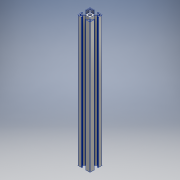
# Autodesk Inventor part: 3030 Extrusion - Y
Saved by Autodesk Inventor 2016 (Build 200138000, 138)
## iProperties
Created: 2016-12-24
Part Number: 3030 Extrusion - Y
Material: Aluminum 6061
Document SubType Name: Modeling
Designer: Scott
Mass: 352.135 g
Surface Area: 1477.59 cm^2
Volume: 130.42 cm^3
Density: 2.7 g/cm^3
Appearance: Aluminum - Flat
Author: Scott
Autodesk Inventor part; units mm, degrees
ref_plane "YZ Plane" through (0, 0, 0) normal (1, 0, 0) x (0, 1, 0)
ref_plane "XZ Plane" through (0, 0, 0) normal (0, 1, 0) x (-1, 0, 0)
ref_plane "XY Plane" through (0, 0, 0) normal (0, 0, 1) x (1, 0, 0)
sketch "Sketch1" plane through (0, 0, 0) normal (0, 0, 1) x (1, 0, 0)
  line L0 (1.9798, -0.0606) -> (9.8798, -0.0606)
  line L1 (20.0798, -0.0606) -> (27.9798, -0.0606)
  arc A0 (-0.0202, 1.9394) -> (1.9798, -0.0606) centre (1.9798, 1.9394) ccw
  line L2 (29.9798, 1.9394) -> (29.9798, 9.8394)
  arc A1 (27.9798, -0.0606) -> (29.9798, 1.9394) centre (27.9798, 1.9394) ccw
  line L3 (29.9798, 20.0394) -> (29.9798, 27.9394)
  arc A2 (29.9798, 27.9394) -> (27.9798, 29.9394) centre (27.9798, 27.9394) ccw
  line L4 (27.9798, 29.9394) -> (20.0798, 29.9394)
  line L5 (9.8798, 29.9394) -> (1.9798, 29.9394)
  line L6 (-0.0202, 27.9394) -> (-0.0202, 20.0394)
  line L7 (-0.0202, 9.8394) -> (-0.0202, 1.9394)
  arc A3 (1.9798, 29.9394) -> (-0.0202, 27.9394) centre (1.9798, 27.9394) ccw
  circle A4 centre (14.9798, 14.9394) radius 3.4
  line L8 (24.9798, 1.4394) -> (27.9798, 1.4394)
  arc A5 (27.9798, 1.4394) -> (28.4798, 1.9394) centre (27.9798, 1.9394) ccw
  line L9 (28.4798, 1.9394) -> (28.4798, 4.9394)
  arc A6 (28.4798, 4.9394) -> (27.9798, 5.4394) centre (27.9798, 4.9394) ccw
  line L10 (29.2298, 9.8394) -> (29.2298, 10.8394)
  line L11 (29.2298, 19.0394) -> (29.2298, 20.0394)
  line L12 (28.4798, 7.1894) -> (28.4798, 10.8394)
  arc A7 (27.9798, 6.6894) -> (28.4798, 7.1894) centre (27.9798, 7.1894) ccw
  line L13 (28.4798, 19.0394) -> (28.4798, 22.6894)
  arc A8 (28.4798, 22.6894) -> (27.9798, 23.1894) centre (27.9798, 22.6894) ccw
  line L14 (20.9262, 19.8252) -> (24.144, 23.0429)
  arc A9 (24.4975, 23.1894) -> (24.144, 23.0429) centre (24.4975, 22.6894) ccw
  line L15 (20.9262, 10.0536) -> (24.144, 6.8358)
  arc A10 (20.7798, 10.4071) -> (20.9262, 10.0536) centre (21.2798, 10.4071) ccw
  line L16 (24.4975, 6.6894) -> (27.9798, 6.6894)
  arc A11 (24.144, 6.8358) -> (24.4975, 6.6894) centre (24.4975, 7.1894) ccw
  line L17 (24.4975, 23.1894) -> (27.9798, 23.1894)
  line L18 (28.4798, 10.8394) -> (29.2298, 10.8394)
  line L19 (28.4798, 19.0394) -> (29.2298, 19.0394)
  line L20 (29.2298, 9.8394) -> (29.9798, 9.8394)
  line L21 (29.2298, 20.0394) -> (29.9798, 20.0394)
  line L22 (20.7798, 10.4071) -> (20.7798, 19.4716)
  arc A12 (20.9262, 19.8252) -> (20.7798, 19.4716) centre (21.2798, 19.4716) ccw
  line L23 (24.4798, 1.9394) -> (24.4798, 4.9394)
  arc A13 (24.4798, 1.9394) -> (24.9798, 1.4394) centre (24.9798, 1.9394) ccw
  line L24 (24.9798, 5.4394) -> (27.9798, 5.4394)
  arc A14 (24.9798, 5.4394) -> (24.4798, 4.9394) centre (24.9798, 4.9394) ccw
  line L25 (28.4798, 24.9394) -> (28.4798, 27.9394)
  arc A15 (28.4798, 27.9394) -> (27.9798, 28.4394) centre (27.9798, 27.9394) ccw
  line L26 (27.9798, 28.4394) -> (24.9798, 28.4394)
  arc A16 (24.9798, 28.4394) -> (24.4798, 27.9394) centre (24.9798, 27.9394) ccw
  line L27 (20.0798, 29.1894) -> (19.0798, 29.1894)
  line L28 (10.8798, 29.1894) -> (9.8798, 29.1894)
  line L29 (22.7298, 28.4394) -> (19.0798, 28.4394)
  arc A17 (23.2298, 27.9394) -> (22.7298, 28.4394) centre (22.7298, 27.9394) ccw
  line L30 (10.8798, 28.4394) -> (7.2298, 28.4394)
  arc A18 (7.2298, 28.4394) -> (6.7298, 27.9394) centre (7.2298, 27.9394) ccw
  line L31 (10.094, 20.8858) -> (6.8762, 24.1036)
  arc A19 (6.7298, 24.4571) -> (6.8762, 24.1036) centre (7.2298, 24.4571) ccw
  line L32 (19.8656, 20.8858) -> (23.0833, 24.1036)
  arc A20 (19.512, 20.7394) -> (19.8656, 20.8858) centre (19.512, 21.2394) ccw
  line L33 (23.2298, 24.4571) -> (23.2298, 27.9394)
  arc A21 (23.0833, 24.1036) -> (23.2298, 24.4571) centre (22.7298, 24.4571) ccw
  line L34 (6.7298, 24.4571) -> (6.7298, 27.9394)
  line L35 (19.0798, 28.4394) -> (19.0798, 29.1894)
  line L36 (10.8798, 28.4394) -> (10.8798, 29.1894)
  line L37 (20.0798, 29.1894) -> (20.0798, 29.9394)
  line L38 (9.8798, 29.1894) -> (9.8798, 29.9394)
  line L39 (19.512, 20.7394) -> (10.4475, 20.7394)
  arc A22 (10.094, 20.8858) -> (10.4475, 20.7394) centre (10.4475, 21.2394) ccw
  line L40 (27.9798, 24.4394) -> (24.9798, 24.4394)
  arc A23 (27.9798, 24.4394) -> (28.4798, 24.9394) centre (27.9798, 24.9394) ccw
  line L41 (24.4798, 24.9394) -> (24.4798, 27.9394)
  arc A24 (24.4798, 24.9394) -> (24.9798, 24.4394) centre (24.9798, 24.9394) ccw
  line L42 (4.9798, 28.4394) -> (1.9798, 28.4394)
  arc A25 (1.9798, 28.4394) -> (1.4798, 27.9394) centre (1.9798, 27.9394) ccw
  line L43 (1.4798, 27.9394) -> (1.4798, 24.9394)
  arc A26 (1.4798, 24.9394) -> (1.9798, 24.4394) centre (1.9798, 24.9394) ccw
  line L44 (0.7298, 20.0394) -> (0.7298, 19.0394)
  line L45 (0.7298, 10.8394) -> (0.7298, 9.8394)
  line L46 (1.4798, 22.6894) -> (1.4798, 19.0394)
  arc A27 (1.9798, 23.1894) -> (1.4798, 22.6894) centre (1.9798, 22.6894) ccw
  line L47 (1.4798, 10.8394) -> (1.4798, 7.1894)
  arc A28 (1.4798, 7.1894) -> (1.9798, 6.6894) centre (1.9798, 7.1894) ccw
  line L48 (9.0333, 10.0536) -> (5.8156, 6.8358)
  arc A29 (5.462, 6.6894) -> (5.8156, 6.8358) centre (5.462, 7.1894) ccw
  line L49 (9.0333, 19.8252) -> (5.8156, 23.0429)
  arc A30 (9.1798, 19.4716) -> (9.0333, 19.8252) centre (8.6798, 19.4716) ccw
  line L50 (5.462, 23.1894) -> (1.9798, 23.1894)
  arc A31 (5.8156, 23.0429) -> (5.462, 23.1894) centre (5.462, 22.6894) ccw
  line L51 (5.462, 6.6894) -> (1.9798, 6.6894)
  line L52 (1.4798, 19.0394) -> (0.7298, 19.0394)
  line L53 (1.4798, 10.8394) -> (0.7298, 10.8394)
  line L54 (0.7298, 20.0394) -> (-0.0202, 20.0394)
  line L55 (0.7298, 9.8394) -> (-0.0202, 9.8394)
  line L56 (9.1798, 19.4716) -> (9.1798, 10.4071)
  arc A32 (9.0333, 10.0536) -> (9.1798, 10.4071) centre (8.6798, 10.4071) ccw
  line L57 (5.4798, 27.9394) -> (5.4798, 24.9394)
  arc A33 (5.4798, 27.9394) -> (4.9798, 28.4394) centre (4.9798, 27.9394) ccw
  line L58 (4.9798, 24.4394) -> (1.9798, 24.4394)
  arc A34 (4.9798, 24.4394) -> (5.4798, 24.9394) centre (4.9798, 24.9394) ccw
  line L59 (1.4798, 4.9394) -> (1.4798, 1.9394)
  arc A35 (1.4798, 1.9394) -> (1.9798, 1.4394) centre (1.9798, 1.9394) ccw
  line L60 (1.9798, 1.4394) -> (4.9798, 1.4394)
  arc A36 (4.9798, 1.4394) -> (5.4798, 1.9394) centre (4.9798, 1.9394) ccw
  line L61 (9.8798, 0.6894) -> (10.8798, 0.6894)
  line L62 (19.0798, 0.6894) -> (20.0798, 0.6894)
  line L63 (7.2298, 1.4394) -> (10.8798, 1.4394)
  arc A37 (6.7298, 1.9394) -> (7.2298, 1.4394) centre (7.2298, 1.9394) ccw
  line L64 (19.0798, 1.4394) -> (22.7298, 1.4394)
  arc A38 (22.7298, 1.4394) -> (23.2298, 1.9394) centre (22.7298, 1.9394) ccw
  line L65 (19.8656, 8.9929) -> (23.0833, 5.7752)
  arc A39 (23.2298, 5.4216) -> (23.0833, 5.7752) centre (22.7298, 5.4216) ccw
  line L66 (10.094, 8.9929) -> (6.8762, 5.7752)
  arc A40 (10.4475, 9.1394) -> (10.094, 8.9929) centre (10.4475, 8.6394) ccw
  line L67 (6.7298, 5.4216) -> (6.7298, 1.9394)
  arc A41 (6.8762, 5.7752) -> (6.7298, 5.4216) centre (7.2298, 5.4216) ccw
  line L68 (23.2298, 5.4216) -> (23.2298, 1.9394)
  line L69 (10.8798, 1.4394) -> (10.8798, 0.6894)
  line L70 (19.0798, 1.4394) -> (19.0798, 0.6894)
  line L71 (9.8798, 0.6894) -> (9.8798, -0.0606)
  line L72 (20.0798, 0.6894) -> (20.0798, -0.0606)
  line L73 (10.4475, 9.1394) -> (19.512, 9.1394)
  arc A42 (19.8656, 8.9929) -> (19.512, 9.1394) centre (19.512, 8.6394) ccw
  line L74 (1.9798, 5.4394) -> (4.9798, 5.4394)
  arc A43 (1.9798, 5.4394) -> (1.4798, 4.9394) centre (1.9798, 4.9394) ccw
  line L75 (5.4798, 4.9394) -> (5.4798, 1.9394)
  arc A44 (5.4798, 4.9394) -> (4.9798, 5.4394) centre (4.9798, 4.9394) ccw
  point P0 (0, 0)
  dimension "d1" = 2
  dimension "d2" = 0.5
  dimension "d3" = 6.8
  dimension "d4" = 45
  dimension "d5" = 45
  dimension "d6" = 45
  dimension "d7" = 90
  dimension "d8" = 90
  dimension "d9" = 90
  dimension "d10" = 90
  dimension "d11" = 90
  dimension "d12" = 90
  dimension "d13" = 45
  dimension "d14" = 45
  dimension "d15" = 90
  dimension "d16" = 90
  dimension "d17" = 90
  dimension "d18" = 90
  dimension "d19" = 90
  dimension "d20" = 90
  dimension "d21" = 90
  dimension "d22" = 90
  dimension "d23" = 90
  dimension "d24" = 90
  dimension "d25" = 90
  dimension "d26" = 90
  dimension "d27" = 90
  dimension "d28" = 90
  dimension "d29" = 90
  dimension "d30" = 90
  dimension "d31" = 90
  dimension "d32" = 90
  dimension "d33" = 90
  dimension "d34" = 90
  dimension "d35" = 90
  dimension "d36" = 90
  dimension "d37" = 90
  dimension "d38" = 90
  dimension "d39" = 90
  dimension "d40" = 90
  dimension "d41" = 90
  dimension "d42" = 90
  dimension "d43" = 90
  dimension "d44" = 90
  dimension "d45" = 0.75
  dimension "d46" = 5.5
  dimension "d47" = 6.75
  dimension "d48" = 9.2
  dimension "d49" = 9.9
  dimension "d50" = 10.9
  dimension "d51" = 19.1
  dimension "d52" = 20.1
  dimension "d53" = 20.8
  dimension "d54" = 23.25
  dimension "d55" = 24.5
  dimension "d56" = 28.5
  dimension "d57" = 29.25
  dimension "d58" = 10.2
  dimension "d59" = 1
  dimension "d60" = 9.2
  dimension "d61" = 8.4
  dimension "d62" = 4.4
  dimension "d63" = 14.6
  dimension "d64" = 18.6
  constraints: 152 end point, 88 point on circle, 88 tangent, 45 centre point, 39 equal radius, 31 parallel, 1 horizontal, 1 perpendicular, 1 vertical
  measures "d1" radius of A2
  measures "d2" radius of A15
  measures "d3" diameter of A4
  measures "d4" angle of L3 L14
  measures "d5" angle of L15 L3
  measures "d6" angle of L65 L3
  measures "d7" angle of L29 L3
  measures "d8" angle of L64 L3
  measures "d9" angle of L28 L3
  measures "d10" angle of L61 L3
  measures "d11" angle of L30 L3
  measures "d12" angle of L63 L3
  measures "d13" angle of L66 L3
  measures "d14" angle of L48 L3
  measures "d15" angle of L5 L3
  measures "d16" angle of L0 L3
  measures "d17" angle of L50 L3
  measures "d18" angle of L51 L3
  measures "d19" angle of L42 L3
  measures "d20" angle of L58 L3
  measures "d21" angle of L74 L3
  measures "d22" angle of L60 L3
  measures "d23" angle of L52 L3
  measures "d24" angle of L53 L3
  measures "d25" angle of L54 L3
  measures "d26" angle of L55 L3
  measures "d27" angle of L21 L2
  measures "d28" angle of L21 L10
  measures "d29" angle of L21 L13
  measures "d30" angle of L21 L12
  measures "d31" angle of L21 L9
  measures "d32" angle of L21 L23
  measures "d33" angle of L21 L68
  measures "d34" angle of L21 L72
  measures "d35" angle of L21 L70
  measures "d36" angle of L21 L69
  measures "d37" angle of L21 L71
  measures "d38" angle of L21 L67
  measures "d39" angle of L21 L75
  measures "d40" angle of L21 L46
  measures "d41" angle of L21 L47
  measures "d42" angle of L21 L59
  measures "d43" angle of L21 L45
  measures "d44" angle of L21 L7
  measures "d45" distance between parallel lines of L11 L3
  measures "d46" distance between parallel lines of L41 L3
  measures "d47" distance between parallel lines of L3 L33
  measures "d48" distance between parallel lines of L3 L22
  measures "d49" distance between parallel lines of L37 L3
  measures "d50" distance between parallel lines of L35 L3
  measures "d51" distance between parallel lines of L36 L3
  measures "d52" distance between parallel lines of L38 L3
  measures "d53" distance between parallel lines of L3 L56
  measures "d54" distance between parallel lines of L3 L34
  measures "d55" distance between parallel lines of L57 L3
  measures "d56" distance between parallel lines of L3 L43
  measures "d57" distance between parallel lines of L44 L3
  measures "d58" distance between parallel lines of L21 L20
  measures "d59" distance between parallel lines of L21 L19
  measures "d60" distance between parallel lines of L21 L18
  measures "d61" distance between parallel lines of L21 L26
  measures "d62" distance between parallel lines of L21 L40
  measures "d63" distance between parallel lines of L21 L24
  measures "d64" distance between parallel lines of L21 L8
extrude "Extrusion1" add sketch "Sketch1" along normal mid plane 320
equation "\"d119\" = frame_depth - 2 * extrusion_size"
equation "\"platform_width\" = 214"
equation "\"platform_depth\" = 214"
equation "\"bed_cl_y_offset\" = 173.25"
equation "\"frame_depth\" = 380"
equation "\"extrusion_size\" = 30"
body "Solid1"
